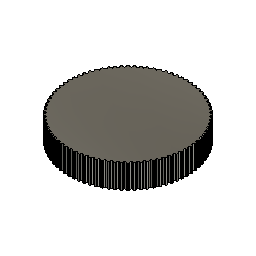
gear_80z (Autodesk Fusion 360 design; units mm, degrees)
Autodesk Fusion 360 part; units mm, degrees
sketch "Sketch1" plane through (0, 0, 0) normal (0, 0, 1) x (1, 0, 0) in component "gt2 pulley"
  circle A0 centre (0, 0) radius 25.4648 construction
  circle A1 centre (0, 0) radius 24.4608 construction
  line L0 (0, 0) -> (0, 25.4648) construction
  line L1 (0, 0) -> (0.9997, 25.4452) construction
  line L2 (0, 0) -> (1.4049, 25.426) construction
  circle A2 centre (0, 0) radius 25.2108 construction
  arc A3 (0.3957, 25.0743) -> (0.4723, 24.7771) centre (1.3909, 25.1724) ccw
  circle A4 centre (0, 0) radius 25.0608 construction
  arc A5 (0.2478, 25.2096) -> (0, 25.2108) centre (0, 0) ccw
  arc A6 (0.3957, 25.0743) -> (0.2478, 25.2096) centre (0.2464, 25.0596) ccw
  arc A7 (0.4723, 24.7771) -> (0.9603, 24.4419) centre (0.9821, 24.9965) ccw
  arc A8 (0, 25.2108) -> (-0.2478, 25.2096) centre (0, 0) ccw
  arc A9 (-0.2478, 25.2096) -> (-0.3957, 25.0743) centre (-0.2464, 25.0596) ccw
  arc A10 (-0.4723, 24.7771) -> (-0.3957, 25.0743) centre (-1.3909, 25.1724) ccw
  arc A11 (-0.9601, 24.4419) -> (-0.4723, 24.7771) centre (-0.9821, 24.9965) ccw
  arc A12 (0.9603, 24.4419) -> (-0.9603, 24.4419) centre (0, 0) ccw
  point P0 (1.3909, 25.1724)
  point P1 (0, 25.2108)
  dimension "d18" = 50.9296
  dimension "d19" = 2.25
  dimension "d22" = 1.004
  dimension "d24" = 0.75
  dimension "d26" = 1
  dimension "d27" = 0.15
  dimension "d28" = 0.15
  dimension "d47" = 0.555
  dimension "d52" = 3.812
  constraint coincident A0.centre A1.centre
  constraint coincident A0 L0.end
  constraint vertical L0
  constraint coincident A0 L1.end
  constraint coincident A0 L2.end
  constraint concentric A1 A2
  constraint coincident A1 A7.end
  constraint coincident L1 A7.end
  constraint coincident A2 P0
  constraint coincident L2 P0
  constraint coincident P0 A3.centre
  constraint coincident A2 P1
  constraint coincident L0 P1
  constraint concentric A2 A4
  constraint coincident P1 A5.end
  constraint coincident A4 A6.centre
  constraint coincident A3.start A6.start
  constraint tangent A3 A6
  constraint tangent A3 A7
  constraint symmetric L0 A7.end A12.end
  constraint symmetric L0 A3.start A9.end
  constraint symmetric L0 A3.end A10.start
  constraint symmetric L0 A3 A10
  constraint symmetric L0 A5.start A8.end
  constraint symmetric L0 P1 A5.end
  constraint symmetric L0 A5 A8
  constraint symmetric L0 A6 A9
  constraint symmetric L0 A7 A11
  constraint coincident A1 A11.start
  constraint tangent A1 A7
  constraint coincident L1 A7.centre
  measures "d18" diameter of A0
  measures "d19" angle of L0 L1
  measures "d22" distance of A0 A1
  measures "d24" distance of A1 A2
  measures "d26" radius of A3
  measures "d27" distance of A2 A4
  measures "d28" radius of A6
  measures "d47" radius of A7
extrude "Extrude1" add sketch "Sketch1" along normal blind 10 makes body 1
pattern_circular "C-Pattern1" count 80 over 360 about axis through (0, 0, 1.75) along (0, 0, 1) of bodies 1 makes body 2 at (-2.0254, 24.3768, 6.6667) makes body 3 at (-3.9318, 24.1427, 6.6667) makes body 4 at (-5.8139, 23.7598, 6.6667) makes body 5 at (-6.8448, 23.4836, 3.3333) makes body 6 at (-8.6662, 22.8742, 3.3333) makes body 7 at (-10.4342, 22.1237, 3.3333) makes body 8 at (-12.1378, 21.2368, 3.3333) makes body 9 at (-14.9752, 19.341, 6.6667) makes body 10 at (-16.2879, 18.2493, 6.6667) makes body 11 at (-16.7601, 17.8165, 3.3333) makes body 12 at (-18.1063, 16.4466, 6.6667) makes body 13 at (-20.2189, 13.7668, 6.6667) makes body 14 at (-20.4562, 13.4117, 3.3333) makes body 15 at (-21.8429, 11.0099, 6.6667) makes body 16 at (-22.3024, 10.0465, 3.3333) makes body 17 at (-23.0219, 8.2657, 3.3333) makes body 18 at (-23.7598, 5.8141, 6.6667) makes body 19 at (-24.1761, 3.7212, 6.6667) makes body 20 at (-24.3935, 1.8129, 6.6667) makes body 21 at (-24.4606, -0.1066, 6.6667) makes body 22 at (-24.4326, -1.1736, 3.3333) makes body 23 at (-24.1427, -3.9318, 6.6667) makes body 24 at (-23.7598, -5.8139, 6.6667) makes body 25 at (-23.4836, -6.8448, 3.3333) makes body 26 at (-22.8742, -8.6662, 3.3333) makes body 27 at (-22.1237, -10.4342, 3.3333) makes body 28 at (-20.8003, -12.8715, 6.6667) makes body 29 at (-19.341, -14.9752, 6.6667) makes body 30 at (-18.2493, -16.2879, 6.6667) makes body 31 at (-16.7603, -17.8164, 6.6667) makes body 32 at (-15.9671, -18.5306, 6.6667) makes body 33 at (-14.2913, -19.8517, 6.6667) makes body 34 at (-13.4117, -20.4562, 3.3333) makes body 35 at (-10.4344, -22.1236, 6.6667) makes body 36 at (-8.6664, -22.8741, 6.6667) makes body 37 at (-8.2657, -23.0219, 3.3333) makes body 38 at (-5.8141, -23.7598, 6.6667) makes body 39 at (-3.7212, -24.1761, 6.6667) makes body 40 at (-1.8129, -24.3935, 6.6667) makes body 41 at (0.1066, -24.4606, 6.6667) makes body 42 at (1.1736, -24.4326, 3.3333) makes body 43 at (3.9318, -24.1427, 6.6667) makes body 44 at (5.8139, -23.7598, 6.6667) makes body 45 at (6.8448, -23.4836, 3.3333) makes body 46 at (8.6662, -22.8742, 3.3333) makes body 47 at (10.4342, -22.1237, 3.3333) makes body 48 at (12.8715, -20.8003, 6.6667) makes body 49 at (14.9752, -19.341, 6.6667) makes body 50 at (16.2879, -18.2493, 6.6667) makes body 51 at (17.6695, -16.9151, 6.6667) makes body 52 at (19.0765, -15.3107, 6.6667) makes body 53 at (19.3409, -14.9753, 3.3333) makes body 54 at (20.4562, -13.4117, 3.3333) makes body 55 at (21.8429, -11.0099, 6.6667) makes body 56 at (22.8741, -8.6664, 6.6667) makes body 57 at (23.0219, -8.2657, 3.3333) makes body 58 at (23.8096, -5.6065, 6.6667) makes body 59 at (24.1761, -3.7212, 6.6667) makes body 60 at (24.4326, -1.1738, 6.6667) makes body 61 at (24.4606, 0.1066, 6.6667) makes body 62 at (24.3768, 2.0254, 6.6667) makes body 63 at (24.1427, 3.9318, 6.6667) makes body 64 at (23.7598, 5.8139, 6.6667) makes body 65 at (23.4836, 6.8448, 3.3333) makes body 66 at (22.8742, 8.6662, 3.3333) makes body 67 at (22.1237, 10.4342, 3.3333) makes body 68 at (20.8003, 12.8715, 6.6667) makes body 69 at (19.8518, 14.2911, 6.6667) makes body 70 at (18.2493, 16.2879, 6.6667) makes body 71 at (17.8165, 16.7601, 3.3333) makes body 72 at (15.9671, 18.5306, 6.6667) makes body 73 at (13.7668, 20.2189, 6.6667) makes body 74 at (13.4117, 20.4562, 3.3333) makes body 75 at (11.0099, 21.8429, 6.6667) makes body 76 at (8.6664, 22.8741, 6.6667) makes body 77 at (6.845, 23.4835, 6.6667) makes body 78 at (5.6065, 23.8096, 6.6667) makes body 79 at (3.7212, 24.1761, 6.6667) makes body 80 at (1.8129, 24.3935, 6.6667)
sketch "Sketch2" plane through (0, 0, 10) normal (0, 0, 1) x (-1, 0, 0)
  arc A0 (-8.1247, -23.7248) -> (-8.0259, -23.8991) centre (-7.9782, -23.7569) ccw
  arc A1 (-8.0259, -23.8991) -> (-7.5545, -24.0523) centre (0, 0) ccw
  arc A2 (-7.5545, -24.0523) -> (-7.372, -23.9693) centre (-7.5095, -23.9092) ccw
  arc A3 (-7.2074, -23.7104) -> (-7.372, -23.9693) centre (-6.4559, -24.3702) ccw
  arc A4 (-6.6398, -23.5424) -> (-7.2074, -23.7104) centre (-6.7903, -24.0766) ccw
  arc A5 (-8.4663, -22.9489) -> (-6.6398, -23.5424) centre (0, 0) ccw
  arc A6 (-8.1057, -23.4185) -> (-8.4663, -22.9489) centre (-8.6584, -23.4696) ccw
  arc A7 (-8.1247, -23.7248) -> (-8.1057, -23.4185) centre (-9.1015, -23.5106) ccw
  circle A8 centre (0, 0) radius 24.4608
  constraint concentric A1 A8
extrude "Extrude2" add sketch "Sketch2" against normal blind 10 contours A5 A8 bodies 1 2 3 4 5 6 7 8 9 10 11 12 13 14 15 16 17 18 19 20 21 22 23 24 25 26 27 28 29 30 31 32 33 34 35 36 37 38 39 40 41 42 43 44 45 46 47 48 49 50 51 52 53 54 55 56 57 58 59 60 61 62 63 64 65 66 67 68 69 70 71 72 73 74 75 76 77 78 79 80
extrude "Extrude4" [suppressed] in component "gt2 pulley"
pattern_circular "C-Pattern7" [suppressed] in component "gt2 pulley"
extrude "Extrude3" [suppressed] in component "gt2 pulley"
pattern_circular "C-Pattern6" [suppressed] in component "gt2 pulley"
extrude "Extrude2'" [suppressed] in component "gt2 pulley"
pattern_circular "C-Pattern5" [suppressed] in component "gt2 pulley"
extrude "Extrude1'" [suppressed] in component "gt2 pulley"
pattern_circular "C-Pattern4" [suppressed] in component "gt2 pulley"
pattern_circular "C-Pattern3" [suppressed] in component "gt2 pulley"
pattern_circular "C-Pattern2" [suppressed] in component "gt2 pulley"
pattern_circular "C-Pattern1'" [suppressed] in component "gt2 pulley"
copy_body "Body->Comp1" [suppressed] in component "Component"
copy_body "Body->Comp2" [suppressed] in component "Component'"
copy_body "Body->Comp3" [suppressed] in component "Component''"
copy_body "Body->Comp4" [suppressed] in component "Component'''"
copy_body "Body->Comp5" [suppressed] in component "Component''''"
copy_body "Body->Comp6" [suppressed] in component "Component'''''"
copy_body "Body->Comp7" [suppressed] in component "Component''''''"
copy_body "Body->Comp8" [suppressed] in component "Component'''''''"
copy_body "Body->Comp9" [suppressed] in component "Component''''''''"
copy_body "Body->Comp10" [suppressed] in component "Component'''''''''"
copy_body "Body->Comp11" [suppressed] in component "Component''''''''''"
copy_body "Body->Comp12" [suppressed] in component "Component'''''''''''"
copy_body "Body->Comp13" [suppressed] in component "Component''''''''''''"
copy_body "Body->Comp14" [suppressed] in component "Component'''''''''''''"
copy_body "Body->Comp15" [suppressed] in component "Component''''''''''''''"
copy_body "Body->Comp16" [suppressed] in component "Component'''''''''''''''"
copy_body "Body->Comp17" [suppressed] in component "Component''''''''''''''''"
copy_body "Body->Comp18" [suppressed] in component "Component'''''''''''''''''"
copy_body "Body->Comp19" [suppressed] in component "Component''''''''''''''''''"
copy_body "Body->Comp20" [suppressed] in component "Component'''''''''''''''''''"
component "gt2 pulley" placed x (1, 0, 0) y (0, 1, 0) z (0, 0, 1) at (0, 0, 0)
equation "NumTeeth = 80" comment "min 20"
equation "ToothPitch = 2 mm"
equation "PullyDia = NumTeeth * ToothPitch / PI"
equation "ToothAng = ( ( 360 / NumTeeth ) * 1 deg )"
equation "TransOffsetAngle = ToothAng * 0.2"
equation "Sholulder_Radius = 0.15 mm"
equation "Root_Radius = 0.555 mm"
equation "TransRadius = 1 mm"
equation "ToolHeight = 0.75 mm"
equation "PLD = 0.254 mm"
equation "d18 = PullyDia"
equation "d19 = ToothAng / 2"
equation "d22 = PLD + ToolHeight"
equation "d24 = ToolHeight"
equation "d26 = TransRadius"
equation "d27 = Sholulder_Radius"
equation "d31 = NumTeeth"
equation "d33 = NumTeeth"
equation "d35 = NumTeeth"
equation "d37 = NumTeeth"
equation "d41 = NumTeeth"
equation "d45 = NumTeeth"
equation "d47 = Root_Radius"
equation "d50 = NumTeeth"
